Autodesk Inventor part; units mm, degrees
(part 4 of 4)
  line L1587 (9.162058, 31.05913) -> (9.162058, 29.329968)
  line L1588 (9.162058, 29.329968) -> (12.322051, 29.331634)
  line L1589 (12.322051, 29.331634) -> (15.482864, 29.334134)
  line L1590 (15.482864, 29.334134) -> (15.485364, 31.06163)
  line L1591 (15.485364, 31.06163) -> (15.48703, 32.788291)
  line L1592 (15.48703, 32.788291) -> (15.003699, 32.788291)
  line L1593 (15.003699, 32.788291) -> (14.520368, 32.788291)
  line L1594 (14.520368, 32.788291) -> (14.520368, 31.559128)
  line L1595 (14.520368, 31.559128) -> (14.520368, 30.329965)
  line L1596 (14.520368, 30.329965) -> (13.674536, 30.329965)
  line L1597 (13.674536, 30.329965) -> (12.828705, 30.329965)
  line L1598 (12.828705, 30.329965) -> (12.827038, 31.386628)
  line L1599 (12.827038, 31.386628) -> (12.824538, 32.442459)
  line L1600 (12.824538, 32.442459) -> (12.345374, 32.442459)
  line L1601 (12.345374, 32.442459) -> (11.86621, 32.442459)
  line L1602 (11.86621, 32.442459) -> (11.86371, 31.386628)
  line L1603 (11.86371, 31.386628) -> (11.862043, 30.329965)
  line L1604 (11.862043, 30.329965) -> (10.99538, 30.329965)
  line L1605 (10.99538, 30.329965) -> (10.128717, 30.329965)
  line L1606 (10.128717, 30.329965) -> (10.128717, 31.559128)
  line L1607 (10.128717, 31.559128) -> (10.128717, 32.788291)
  line L1608 (10.128717, 32.788291) -> (9.645386, 32.788291)
  line L1609 (9.645386, 32.788291) -> (9.162055, 32.788291)
  line L1610 (9.162055, 32.788291) -> (9.162055, 31.059129)
  line L1611 (9.162055, 31.059129) -> (9.162058, 31.05913)
  line L1612 (9.163727, 35.106681) -> (9.16206, 33.188354)
  line L1613 (9.16206, 33.188354) -> (9.641225, 33.188354)
  line L1614 (9.641225, 33.188354) -> (10.120389, 33.188354)
  line L1615 (10.120389, 33.188354) -> (10.120389, 33.90085)
  line L1616 (10.120389, 33.90085) -> (10.120389, 34.613346)
  line L1617 (10.120389, 34.613346) -> (12.803713, 34.613346)
  line L1618 (12.803713, 34.613346) -> (15.487036, 34.613346)
  line L1619 (15.487036, 34.613346) -> (15.48537, 35.111679)
  line L1620 (15.48537, 35.111679) -> (15.48287, 35.609177)
  line L1621 (15.48287, 35.609177) -> (12.802044, 35.611677)
  line L1622 (12.802044, 35.611677) -> (10.120386, 35.613344)
  line L1623 (10.120386, 35.613344) -> (10.120386, 36.321676)
  line L1624 (10.120386, 36.321676) -> (10.120386, 37.030009)
  line L1625 (10.120386, 37.030009) -> (9.643722, 37.028342)
  line L1626 (9.643722, 37.028342) -> (9.166224, 37.025842)
  line L1627 (9.166224, 37.025842) -> (9.163724, 35.106681)
  line L1628 (9.163724, 35.106681) -> (9.163727, 35.106681)
  line L1629 (5.977339, 133.568916) -> (5.975994, 133.167035)
  line L1630 (5.975994, 133.167035) -> (5.984059, 133.164347)
  line L1631 (5.984059, 133.164347) -> (5.992795, 133.160986)
  line L1632 (5.992795, 133.160986) -> (8.5331, 133.16233)
  line L1633 (8.5331, 133.16233) -> (11.073405, 133.164347)
  line L1634 (11.073405, 133.164347) -> (11.075421, 134.540013)
  line L1635 (11.075421, 134.540013) -> (11.076765, 135.916353)
  line L1636 (11.076765, 135.916353) -> (10.686982, 135.916353)
  line L1637 (10.686982, 135.916353) -> (10.297199, 135.916353)
  line L1638 (10.297199, 135.916353) -> (10.297199, 134.945255)
  line L1639 (10.297199, 134.945255) -> (10.297199, 133.974157)
  line L1640 (10.297199, 133.974157) -> (8.138603, 133.972813)
  line L1641 (8.138603, 133.972813) -> (5.979336, 133.970797)
  line L1642 (5.979336, 133.970797) -> (5.97732, 133.568915)
  line L1643 (5.97732, 133.568915) -> (5.977339, 133.568916)
  line L1644 (5.977339, 136.912318) -> (5.975994, 136.507076)
  line L1645 (5.975994, 136.507076) -> (5.984059, 136.504388)
  line L1646 (5.984059, 136.504388) -> (5.992795, 136.501028)
  line L1647 (5.992795, 136.501028) -> (8.5331, 136.502372)
  line L1648 (8.5331, 136.502372) -> (11.073405, 136.504388)
  line L1649 (11.073405, 136.504388) -> (11.073405, 136.910974)
  line L1650 (11.073405, 136.910974) -> (11.073405, 137.317559)
  line L1651 (11.073405, 137.317559) -> (8.526369, 137.317559)
  line L1652 (8.526369, 137.317559) -> (5.979333, 137.317559)
  line L1653 (5.979333, 137.317559) -> (5.977317, 136.912317)
  line L1654 (5.977317, 136.912317) -> (5.977339, 136.912318)
  line L1655 (5.975992, 138.590496) -> (5.975992, 138.201383)
  line L1656 (5.975992, 138.201383) -> (8.523028, 138.201383)
  line L1657 (8.523028, 138.201383) -> (11.070064, 138.201383)
  line L1658 (11.070064, 138.201383) -> (11.070064, 138.584446)
  line L1659 (11.070064, 138.584446) -> (11.070064, 138.967508)
  line L1660 (11.070064, 138.967508) -> (9.334855, 138.968852)
  line L1661 (9.334855, 138.968852) -> (7.598974, 138.970868)
  line L1662 (7.598974, 138.970868) -> (9.334855, 139.790758)
  line L1663 (9.334855, 139.790758) -> (11.070064, 140.609976)
  line L1664 (11.070064, 140.609976) -> (11.070064, 141.001776)
  line L1665 (11.070064, 141.001776) -> (11.070064, 141.393576)
  line L1666 (11.070064, 141.393576) -> (8.523028, 141.393576)
  line L1667 (8.523028, 141.393576) -> (5.975992, 141.393576)
  line L1668 (5.975992, 141.393576) -> (5.977336, 141.00917)
  line L1669 (5.977336, 141.00917) -> (5.979353, 140.624091)
  line L1670 (5.979353, 140.624091) -> (7.755557, 140.620731)
  line L1671 (7.755557, 140.620731) -> (9.531088, 140.617371)
  line L1672 (9.531088, 140.617371) -> (7.75354, 139.798152)
  line L1673 (7.75354, 139.798152) -> (5.975992, 138.978933)
  line L1674 (5.975992, 138.978933) -> (5.975992, 138.590494)
  line L1675 (5.975992, 138.590494) -> (5.975992, 138.590496)
  line L1676 (5.975992, 143.705294) -> (5.975992, 142.313499)
  line L1677 (5.975992, 142.313499) -> (5.984057, 142.31081)
  line L1678 (5.984057, 142.31081) -> (5.992793, 142.30745)
  line L1679 (5.992793, 142.30745) -> (8.533098, 142.308794)
  line L1680 (8.533098, 142.308794) -> (11.073403, 142.31081)
  line L1681 (11.073403, 142.31081) -> (11.075419, 143.703952)
  line L1682 (11.075419, 143.703952) -> (11.076763, 145.096421)
  line L1683 (11.076763, 145.096421) -> (10.68698, 145.096421)
  line L1684 (10.68698, 145.096421) -> (10.297197, 145.096421)
  line L1685 (10.297197, 145.096421) -> (10.297197, 144.108521)
  line L1686 (10.297197, 144.108521) -> (10.297197, 143.120621)
  line L1687 (10.297197, 143.120621) -> (9.615074, 143.120621)
  line L1688 (9.615074, 143.120621) -> (8.932952, 143.120621)
  line L1689 (8.932952, 143.120621) -> (8.932952, 143.970751)
  line L1690 (8.932952, 143.970751) -> (8.932952, 144.820882)
  line L1691 (8.932952, 144.820882) -> (8.543169, 144.820882)
  line L1692 (8.543169, 144.820882) -> (8.153386, 144.820882)
  line L1693 (8.153386, 144.820882) -> (8.153386, 143.970751)
  line L1694 (8.153386, 143.970751) -> (8.153386, 143.120621)
  line L1695 (8.153386, 143.120621) -> (7.454464, 143.120621)
  line L1696 (7.454464, 143.120621) -> (6.755542, 143.120621)
  line L1697 (6.755542, 143.120621) -> (6.755542, 144.108521)
  line L1698 (6.755542, 144.108521) -> (6.755542, 145.096421)
  line L1699 (6.755542, 145.096421) -> (6.365759, 145.096421)
  line L1700 (6.365759, 145.096421) -> (5.975976, 145.096421)
  line L1701 (5.975976, 145.096421) -> (5.975976, 143.705296)
  line L1702 (5.975976, 143.705296) -> (5.975992, 143.705294)
  line L1703 (5.977339, 148.867844) -> (5.975994, 147.488817)
  line L1704 (5.975994, 147.488817) -> (8.524376, 147.490161)
  line L1705 (8.524376, 147.490161) -> (11.073419, 147.492177)
  line L1706 (11.073419, 147.492177) -> (11.075435, 147.893386)
  line L1707 (11.075435, 147.893386) -> (11.076779, 148.295267)
  line L1708 (11.076779, 148.295267) -> (10.025036, 148.295267)
  line L1709 (10.025036, 148.295267) -> (8.973293, 148.295267)
  line L1710 (8.973293, 148.295267) -> (8.973293, 149.131958)
  line L1711 (8.973293, 149.131958) -> (8.973293, 149.968649)
  line L1712 (8.973293, 149.968649) -> (8.58687, 149.968649)
  line L1713 (8.58687, 149.968649) -> (8.200447, 149.968649)
  line L1714 (8.200447, 149.968649) -> (8.200447, 149.131958)
  line L1715 (8.200447, 149.131958) -> (8.200447, 148.295267)
  line L1716 (8.200447, 148.295267) -> (7.474642, 148.295267)
  line L1717 (7.474642, 148.295267) -> (6.748837, 148.295267)
  line L1718 (6.748837, 148.295267) -> (6.748837, 149.273086)
  line L1719 (6.748837, 149.273086) -> (6.748837, 150.250904)
  line L1720 (6.748837, 150.250904) -> (6.364431, 150.24956)
  line L1721 (6.364431, 150.24956) -> (5.979352, 150.247544)
  line L1722 (5.979352, 150.247544) -> (5.977336, 148.867844)
  line L1723 (5.977336, 148.867844) -> (5.977339, 148.867844)
  line L1724 (5.975992, 155.076112) -> (5.975992, 154.672887)
  line L1725 (5.975992, 154.672887) -> (8.526381, 154.672887)
  line L1726 (8.526381, 154.672887) -> (11.07677, 154.672887)
  line L1727 (11.07677, 154.672887) -> (11.075425, 156.049227)
  line L1728 (11.075425, 156.049227) -> (11.073409, 157.424893)
  line L1729 (11.073409, 157.424893) -> (10.686986, 157.424893)
  line L1730 (10.686986, 157.424893) -> (10.300564, 157.424893)
  line L1731 (10.300564, 157.424893) -> (10.298547, 156.452449)
  line L1732 (10.298547, 156.452449) -> (10.297203, 155.479335)
  line L1733 (10.297203, 155.479335) -> (8.136593, 155.479335)
  line L1734 (8.136593, 155.479335) -> (5.975983, 155.479335)
  line L1735 (5.975983, 155.479335) -> (5.975983, 155.07611)
  line L1736 (5.975983, 155.07611) -> (5.975992, 155.076112)
  line L1737 (5.975992, 158.449994) -> (5.975992, 158.046769)
  line L1738 (5.975992, 158.046769) -> (8.526381, 158.046769)
  line L1739 (8.526381, 158.046769) -> (11.07677, 158.046769)
  line L1740 (11.07677, 158.046769) -> (11.075425, 159.423109)
  line L1741 (11.075425, 159.423109) -> (11.073409, 160.798775)
  line L1742 (11.073409, 160.798775) -> (10.686986, 160.798775)
  line L1743 (10.686986, 160.798775) -> (10.300564, 160.798775)
  line L1744 (10.300564, 160.798775) -> (10.298547, 159.826331)
  line L1745 (10.298547, 159.826331) -> (10.297203, 158.853217)
  line L1746 (10.297203, 158.853217) -> (8.136593, 158.853217)
  line L1747 (8.136593, 158.853217) -> (5.975983, 158.853217)
  line L1748 (5.975983, 158.853217) -> (5.975983, 158.449992)
  line L1749 (5.975983, 158.449992) -> (5.975992, 158.449994)
  line L1750 (5.975992, 165.199282) -> (5.975992, 164.785976)
  line L1751 (5.975992, 164.785976) -> (5.990777, 164.789336)
  line L1752 (5.990777, 164.789336) -> (6.006234, 164.793368)
  line L1753 (6.006234, 164.793368) -> (8.524372, 165.260436)
  line L1754 (8.524372, 165.260436) -> (11.043181, 165.728177)
  line L1755 (11.043181, 165.728177) -> (11.059982, 165.732209)
  line L1756 (11.059982, 165.732209) -> (11.076783, 165.736242)
  line L1757 (11.076783, 165.736242) -> (11.076783, 166.134763)
  line L1758 (11.076783, 166.134763) -> (11.076783, 166.533283)
  line L1759 (11.076783, 166.533283) -> (11.064686, 166.535972)
  line L1760 (11.064686, 166.535972) -> (11.053262, 166.53866)
  line L1761 (11.053262, 166.53866) -> (9.337543, 166.917691)
  line L1762 (9.337543, 166.917691) -> (7.621823, 167.297393)
  line L1763 (7.621823, 167.297393) -> (7.677603, 167.308818)
  line L1764 (7.677603, 167.308818) -> (7.733382, 167.320915)
  line L1765 (7.733382, 167.320915) -> (9.402731, 167.670376)
  line L1766 (9.402731, 167.670376) -> (11.07208, 168.019836)
  line L1767 (11.07208, 168.019836) -> (11.074768, 168.021853)
  line L1768 (11.074768, 168.021853) -> (11.076784, 168.024541)
  line L1769 (11.076784, 168.024541) -> (11.07544, 168.423732)
  line L1770 (11.07544, 168.423732) -> (11.073424, 168.822924)
  line L1771 (11.073424, 168.822924) -> (8.529741, 169.294025)
  line L1772 (8.529741, 169.294025) -> (5.986058, 169.765126)
  line L1773 (5.986058, 169.765126) -> (5.981354, 169.762438)
  line L1774 (5.981354, 169.762438) -> (5.975978, 169.75975)
  line L1775 (5.975978, 169.75975) -> (5.975978, 169.350477)
  line L1776 (5.975978, 169.350477) -> (5.975978, 168.941878)
  line L1777 (5.975978, 168.941878) -> (5.994795, 168.937846)
  line L1778 (5.994795, 168.937846) -> (6.01294, 168.933813)
  line L1779 (6.01294, 168.933813) -> (7.829467, 168.658277)
  line L1780 (7.829467, 168.658277) -> (9.64532, 168.38274)
  line L1781 (9.64532, 168.38274) -> (9.660105, 168.381396)
  line L1782 (9.660105, 168.381396) -> (9.675562, 168.37938)
  line L1783 (9.675562, 168.37938) -> (7.825434, 167.979515)
  line L1784 (7.825434, 167.979515) -> (5.975978, 167.579651)
  line L1785 (5.975978, 167.579651) -> (5.975978, 167.27656)
  line L1786 (5.975978, 167.27656) -> (5.975978, 166.972796)
  line L1787 (5.975978, 166.972796) -> (5.994795, 166.969436)
  line L1788 (5.994795, 166.969436) -> (6.012941, 166.965404)
  line L1789 (6.012941, 166.965404) -> (7.82073, 166.574947)
  line L1790 (7.82073, 166.574947) -> (9.628519, 166.184491)
  line L1791 (9.628519, 166.184491) -> (9.650696, 166.179787)
  line L1792 (9.650696, 166.179787) -> (9.672874, 166.175082)
  line L1793 (9.672874, 166.175082) -> (7.863068, 165.900219)
  line L1794 (7.863068, 165.900219) -> (6.053262, 165.625355)
  line L1795 (6.053262, 165.625355) -> (6.014956, 165.619307)
  line L1796 (6.014956, 165.619307) -> (5.975977, 165.612587)
  line L1797 (5.975977, 165.612587) -> (5.975977, 165.19928)
  line L1798 (5.975977, 165.19928) -> (5.975992, 165.199282)
  line L1799 (5.975992, 171.692538) -> (5.975992, 170.298053)
  line L1800 (5.975992, 170.298053) -> (8.526381, 170.298053)
  line L1801 (8.526381, 170.298053) -> (11.07677, 170.298053)
  line L1802 (11.07677, 170.298053) -> (11.07677, 171.692538)
  line L1803 (11.07677, 171.692538) -> (11.07677, 173.087023)
  line L1804 (11.07677, 173.087023) -> (10.686986, 173.087023)
  line L1805 (10.686986, 173.087023) -> (10.297203, 173.087023)
  line L1806 (10.297203, 173.087023) -> (10.297203, 172.095763)
  line L1807 (10.297203, 172.095763) -> (10.297203, 171.104503)
  line L1808 (10.297203, 171.104503) -> (9.615081, 171.104503)
  line L1809 (9.615081, 171.104503) -> (8.932959, 171.104503)
  line L1810 (8.932959, 171.104503) -> (8.932959, 171.954633)
  line L1811 (8.932959, 171.954633) -> (8.932959, 172.804763)
  line L1812 (8.932959, 172.804763) -> (8.543175, 172.804763)
  line L1813 (8.543175, 172.804763) -> (8.153392, 172.804763)
  line L1814 (8.153392, 172.804763) -> (8.153392, 171.954633)
  line L1815 (8.153392, 171.954633) -> (8.153392, 171.104503)
  line L1816 (8.153392, 171.104503) -> (7.45447, 171.104503)
  line L1817 (7.45447, 171.104503) -> (6.755549, 171.104503)
  line L1818 (6.755549, 171.104503) -> (6.755549, 172.095763)
  line L1819 (6.755549, 172.095763) -> (6.755549, 173.087023)
  line L1820 (6.755549, 173.087023) -> (6.365765, 173.087023)
  line L1821 (6.365765, 173.087023) -> (5.975982, 173.087023)
  line L1822 (5.975982, 173.087023) -> (5.975982, 171.692538)
  line L1823 (5.975982, 171.692538) -> (5.975992, 171.692538)
  line L1824 (5.977339, 174.71463) -> (5.975994, 173.79259)
  line L1825 (5.975994, 173.79259) -> (8.52303, 173.79259)
  line L1826 (8.52303, 173.79259) -> (11.070066, 173.79259)
  line L1827 (11.070066, 173.79259) -> (11.070066, 174.195815)
  line L1828 (11.070066, 174.195815) -> (11.070066, 174.59904)
  line L1829 (11.070066, 174.59904) -> (10.008242, 174.59904)
  line L1830 (10.008242, 174.59904) -> (8.946418, 174.59904)
  line L1831 (8.946418, 174.59904) -> (8.947762, 174.909522)
  line L1832 (8.947762, 174.909522) -> (8.949778, 175.220677)
  line L1833 (8.949778, 175.220677) -> (10.009585, 175.660191)
  line L1834 (10.009585, 175.660191) -> (11.070066, 176.100378)
  line L1835 (11.070066, 176.100378) -> (11.070066, 176.562742)
  line L1836 (11.070066, 176.562742) -> (11.070066, 177.025105)
  line L1837 (11.070066, 177.025105) -> (11.03512, 177.009649)
  line L1838 (11.03512, 177.009649) -> (10.999502, 176.99352)
  line L1839 (10.999502, 176.99352) -> (9.924909, 176.521748)
  line L1840 (9.924909, 176.521748) -> (8.850316, 176.049976)
  line L1841 (8.850316, 176.049976) -> (8.846284, 176.057368)
  line L1842 (8.846284, 176.057368) -> (8.842252, 176.064088)
  line L1843 (8.842252, 176.064088) -> (8.82209, 176.113148)
  line L1844 (8.82209, 176.113148) -> (8.801257, 176.161535)
  line L1845 (8.801257, 176.161535) -> (8.777736, 176.207905)
  line L1846 (8.777736, 176.207905) -> (8.754214, 176.254276)
  line L1847 (8.754214, 176.254276) -> (8.710532, 176.318792)
  line L1848 (8.710532, 176.318792) -> (8.667521, 176.382636)
  line L1849 (8.667521, 176.382636) -> (8.617118, 176.43976)
  line L1850 (8.617118, 176.43976) -> (8.566715, 176.496883)
  line L1851 (8.566715, 176.496883) -> (8.502871, 176.549302)
  line L1852 (8.502871, 176.549302) -> (8.439027, 176.601722)
  line L1853 (8.439027, 176.601722) -> (8.394, 176.631963)
  line L1854 (8.394, 176.631963) -> (8.348302, 176.662205)
  line L1855 (8.348302, 176.662205) -> (8.259592, 176.705216)
  line L1856 (8.259592, 176.705216) -> (8.170211, 176.748226)
  line L1857 (8.170211, 176.748226) -> (8.089566, 176.773764)
  line L1858 (8.089566, 176.773764) -> (8.008921, 176.799302)
  line L1859 (8.008921, 176.799302) -> (7.924916, 176.815431)
  line L1860 (7.924916, 176.815431) -> (7.840911, 176.83156)
  line L1861 (7.840911, 176.83156) -> (7.753545, 176.838952)
  line L1862 (7.753545, 176.838952) -> (7.66618, 176.845672)
  line L1863 (7.66618, 176.845672) -> (7.383922, 176.842312)
  line L1864 (7.383922, 176.842312) -> (7.101665, 176.83828)
  line L1865 (7.101665, 176.83828) -> (7.023708, 176.824167)
  line L1866 (7.023708, 176.824167) -> (6.945752, 176.809382)
  line L1867 (6.945752, 176.809382) -> (6.88258, 176.792581)
  line L1868 (6.88258, 176.792581) -> (6.819408, 176.775108)
  line L1869 (6.819408, 176.775108) -> (6.765645, 176.756291)
  line L1870 (6.765645, 176.756291) -> (6.711882, 176.737474)
  line L1871 (6.711882, 176.737474) -> (6.627876, 176.693791)
  line L1872 (6.627876, 176.693791) -> (6.543871, 176.650109)
  line L1873 (6.543871, 176.650109) -> (6.486748, 176.61113)
  line L1874 (6.486748, 176.61113) -> (6.429624, 176.57148)
  line L1875 (6.429624, 176.57148) -> (6.342259, 176.484114)
  line L1876 (6.342259, 176.484114) -> (6.254893, 176.396749)
  line L1877 (6.254893, 176.396749) -> (6.20449, 176.319465)
  line L1878 (6.20449, 176.319465) -> (6.154087, 176.24218)
  line L1879 (6.154087, 176.24218) -> (6.123174, 176.178336)
  line L1880 (6.123174, 176.178336) -> (6.09226, 176.114492)
  line L1881 (6.09226, 176.114492) -> (6.074787, 176.067449)
  line L1882 (6.074787, 176.067449) -> (6.057314, 176.020406)
  line L1883 (6.057314, 176.020406) -> (6.039841, 175.963283)
  line L1884 (6.039841, 175.963283) -> (6.022368, 175.906159)
  line L1885 (6.022368, 175.906159) -> (6.008927, 175.835595)
  line L1886 (6.008927, 175.835595) -> (5.995486, 175.765031)
  line L1887 (5.995486, 175.765031) -> (5.987421, 175.701187)
  line L1888 (5.987421, 175.701187) -> (5.979357, 175.637343)
  line L1889 (5.979357, 175.637343) -> (5.977341, 174.714632)
  line L1890 (5.977341, 174.714632) -> (5.977339, 174.71463)
  line L1891 (6.750184, 175.097693) -> (6.752872, 175.597018)
  line L1892 (6.752872, 175.597018) -> (6.764297, 175.637341)
  line L1893 (6.764297, 175.637341) -> (6.775722, 175.677663)
  line L1894 (6.775722, 175.677663) -> (6.802603, 175.731427)
  line L1895 (6.802603, 175.731427) -> (6.828813, 175.78519)
  line L1896 (6.828813, 175.78519) -> (6.863759, 175.825512)
  line L1897 (6.863759, 175.825512) -> (6.899377, 175.865835)
  line L1898 (6.899377, 175.865835) -> (6.929619, 175.890028)
  line L1899 (6.929619, 175.890028) -> (6.960533, 175.91355)
  line L1900 (6.960533, 175.91355) -> (6.997495, 175.935055)
  line L1901 (6.997495, 175.935055) -> (7.034457, 175.955888)
  line L1902 (7.034457, 175.955888) -> (7.096957, 175.976049)
  line L1903 (7.096957, 175.976049) -> (7.158785, 175.996883)
  line L1904 (7.158785, 175.996883) -> (7.211204, 176.004275)
  line L1905 (7.211204, 176.004275) -> (7.262951, 176.011668)
  line L1906 (7.262951, 176.011668) -> (7.498166, 176.008307)
  line L1907 (7.498166, 176.008307) -> (7.73338, 176.005619)
  line L1908 (7.73338, 176.005619) -> (7.790503, 175.991506)
  line L1909 (7.790503, 175.991506) -> (7.847627, 175.976721)
  line L1910 (7.847627, 175.976721) -> (7.910127, 175.945136)
  line L1911 (7.910127, 175.945136) -> (7.973299, 175.91355)
  line L1912 (7.973299, 175.91355) -> (8.025046, 175.863147)
  line L1913 (8.025046, 175.863147) -> (8.076121, 175.812072)
  line L1914 (8.076121, 175.812072) -> (8.101659, 175.768389)
  line L1915 (8.101659, 175.768389) -> (8.127196, 175.724706)
  line L1916 (8.127196, 175.724706) -> (8.142653, 175.674303)
  line L1917 (8.142653, 175.674303) -> (8.158782, 175.6239)
  line L1918 (8.158782, 175.6239) -> (8.166175, 175.565433)
  line L1919 (8.166175, 175.565433) -> (8.173567, 175.506293)
  line L1920 (8.173567, 175.506293) -> (8.173567, 175.052664)
  line L1921 (8.173567, 175.052664) -> (8.173567, 174.599036)
  line L1922 (8.173567, 174.599036) -> (7.461204, 174.599036)
  line L1923 (7.461204, 174.599036) -> (6.748167, 174.599036)
  line L1924 (6.748167, 174.599036) -> (6.750183, 175.097691)
  line L1925 (6.750183, 175.097691) -> (6.750184, 175.097693)
  line L1926 (5.977339, 179.835524) -> (5.975994, 179.430955)
  line L1927 (5.975994, 179.430955) -> (8.524376, 179.432299)
  line L1928 (8.524376, 179.432299) -> (11.073419, 179.434316)
  line L1929 (11.073419, 179.434316) -> (11.075435, 180.809982)
  line L1930 (11.075435, 180.809982) -> (11.076779, 182.186322)
  line L1931 (11.076779, 182.186322) -> (10.686996, 182.186322)
  line L1932 (10.686996, 182.186322) -> (10.297212, 182.186322)
  line L1933 (10.297212, 182.186322) -> (10.297212, 181.215224)
  line L1934 (10.297212, 181.215224) -> (10.297212, 180.244126)
  line L1935 (10.297212, 180.244126) -> (8.138616, 180.242782)
  line L1936 (8.138616, 180.242782) -> (5.97935, 180.240766)
  line L1937 (5.97935, 180.240766) -> (5.977333, 179.835524)
  line L1938 (5.977333, 179.835524) -> (5.977339, 179.835524)
  line L1939 (5.975992, 184.371202) -> (5.975992, 184.064751)
  line L1940 (5.975992, 184.064751) -> (8.518329, 183.289215)
  line L1941 (8.518329, 183.289215) -> (11.05998, 182.51368)
  line L1942 (11.05998, 182.51368) -> (11.066701, 182.513008)
  line L1943 (11.066701, 182.513008) -> (11.073421, 182.512336)
  line L1944 (11.073421, 182.512336) -> (11.075437, 182.937064)
  line L1945 (11.075437, 182.937064) -> (11.076781, 183.361793)
  line L1946 (11.076781, 183.361793) -> (11.051916, 183.368513)
  line L1947 (11.051916, 183.368513) -> (11.026378, 183.375234)
  line L1948 (11.026378, 183.375234) -> (10.571406, 183.498217)
  line L1949 (10.571406, 183.498217) -> (10.115763, 183.621201)
  line L1950 (10.115763, 183.621201) -> (10.117779, 184.373213)
  line L1951 (10.117779, 184.373213) -> (10.119123, 185.125226)
  line L1952 (10.119123, 185.125226) -> (10.596272, 185.254258)
  line L1953 (10.596272, 185.254258) -> (11.073421, 185.383962)
  line L1954 (11.073421, 185.383962) -> (11.075437, 185.80869)
  line L1955 (11.075437, 185.80869) -> (11.076781, 186.233419)
  line L1956 (11.076781, 186.233419) -> (11.058636, 186.228715)
  line L1957 (11.058636, 186.228715) -> (11.040491, 186.224682)
  line L1958 (11.040491, 186.224682) -> (8.565365, 185.468636)
  line L1959 (8.565365, 185.468636) -> (6.090239, 184.713263)
  line L1960 (6.090239, 184.713263) -> (6.033116, 184.69579)
  line L1961 (6.033116, 184.69579) -> (5.975992, 184.678317)
  line L1962 (5.975992, 184.678317) -> (5.975992, 184.371195)
  line L1963 (5.975992, 184.371195) -> (5.975992, 184.371202)
  line L1964 (8.328807, 184.639347) -> (9.312676, 184.906819)
  line L1965 (9.312676, 184.906819) -> (9.330821, 184.911524)
  line L1966 (9.330821, 184.911524) -> (9.349638, 184.916228)
  line L1967 (9.349638, 184.916228) -> (9.349638, 184.374563)
  line L1968 (9.349638, 184.374563) -> (9.349638, 183.832898)
  line L1969 (9.349638, 183.832898) -> (9.342246, 183.832898)
  line L1970 (9.342246, 183.832898) -> (9.334853, 183.832898)
  line L1971 (9.334853, 183.832898) -> (8.362409, 184.094993)
  line L1972 (8.362409, 184.094993) -> (7.390638, 184.357761)
  line L1973 (7.390638, 184.357761) -> (7.367789, 184.365153)
  line L1974 (7.367789, 184.365153) -> (7.344268, 184.372546)
  line L1975 (7.344268, 184.372546) -> (8.328807, 184.639345)
  line L1976 (8.328807, 184.639345) -> (8.328807, 184.639347)
  line L1977 (5.977339, 187.671678) -> (5.975994, 186.783239)
  line L1978 (5.975994, 186.783239) -> (8.526383, 186.783239)
  line L1979 (8.526383, 186.783239) -> (11.076772, 186.783239)
  line L1980 (11.076772, 186.783239) -> (11.076772, 187.186464)
  line L1981 (11.076772, 187.186464) -> (11.076772, 187.589689)
  line L1982 (11.076772, 187.589689) -> (10.089545, 187.589689)
  line L1983 (10.089545, 187.589689) -> (9.102318, 187.589689)
  line L1984 (9.102318, 187.589689) -> (9.098958, 188.105817)
  line L1985 (9.098958, 188.105817) -> (9.095597, 188.621272)
  line L1986 (9.095597, 188.621272) -> (9.084845, 188.695869)
  line L1987 (9.084845, 188.695869) -> (9.07342, 188.769793)
  line L1988 (9.07342, 188.769793) -> (9.057291, 188.845062)
  line L1989 (9.057291, 188.845062) -> (9.04049, 188.92033)
  line L1990 (9.04049, 188.92033) -> (9.014952, 188.992911)
  line L1991 (9.014952, 188.992911) -> (8.989415, 189.064819)
  line L1992 (8.989415, 189.064819) -> (8.962533, 189.122615)
  line L1993 (8.962533, 189.122615) -> (8.936324, 189.18041)
  line L1994 (8.936324, 189.18041) -> (8.896001, 189.245598)
  line L1995 (8.896001, 189.245598) -> (8.855679, 189.310786)
  line L1996 (8.855679, 189.310786) -> (8.811996, 189.365894)
  line L1997 (8.811996, 189.365894) -> (8.768313, 189.420329)
  line L1998 (8.768313, 189.420329) -> (8.715894, 189.471404)
  line L1999 (8.715894, 189.471404) -> (8.663475, 189.521807)
  line L2000 (8.663475, 189.521807) -> (8.632561, 189.546)
  line L2001 (8.632561, 189.546) -> (8.602319, 189.570866)
  line L2002 (8.602319, 189.570866) -> (8.543852, 189.609172)
  line L2003 (8.543852, 189.609172) -> (8.486056, 189.646806)
  line L2004 (8.486056, 189.646806) -> (8.417508, 189.680408)
  line L2005 (8.417508, 189.680408) -> (8.34896, 189.71401)
  line L2006 (8.34896, 189.71401) -> (8.256218, 189.744252)
  line L2007 (8.256218, 189.744252) -> (8.163476, 189.774494)
  line L2008 (8.163476, 189.774494) -> (8.092912, 189.788607)
  line L2009 (8.092912, 189.788607) -> (8.022348, 189.802047)
  line L2010 (8.022348, 189.802047) -> (7.961864, 189.810112)
  line L2011 (7.961864, 189.810112) -> (7.90138, 189.817504)
  line L2012 (7.90138, 189.817504) -> (7.525039, 189.816832)
  line L2013 (7.525039, 189.816832) -> (7.148697, 189.815488)
  line L2014 (7.148697, 189.815488) -> (7.078133, 189.804063)
  line L2015 (7.078133, 189.804063) -> (7.007569, 189.791967)
  line L2016 (7.007569, 189.791967) -> (6.96523, 189.78323)
  line L2017 (6.96523, 189.78323) -> (6.923564, 189.773822)
  line L2018 (6.923564, 189.773822) -> (6.864424, 189.756349)
  line L2019 (6.864424, 189.756349) -> (6.805957, 189.739548)
  line L2020 (6.805957, 189.739548) -> (6.751521, 189.71737)
  line L2021 (6.751521, 189.71737) -> (6.697086, 189.695193)
  line L2022 (6.697086, 189.695193) -> (6.638619, 189.665623)
  line L2023 (6.638619, 189.665623) -> (6.579479, 189.636053)
  line L2024 (6.579479, 189.636053) -> (6.514963, 189.59237)
  line L2025 (6.514963, 189.59237) -> (6.449775, 189.548688)
  line L2026 (6.449775, 189.548688) -> (6.399372, 189.504333)
  line L2027 (6.399372, 189.504333) -> (6.348969, 189.459978)
  line L2028 (6.348969, 189.459978) -> (6.308646, 189.414951)
  line L2029 (6.308646, 189.414951) -> (6.268324, 189.370597)
  line L2030 (6.268324, 189.370597) -> (6.23069, 189.319522)
  line L2031 (6.23069, 189.319522) -> (6.193727, 189.268446)
  line L2032 (6.193727, 189.268446) -> (6.158781, 189.207291)
  line L2033 (6.158781, 189.207291) -> (6.123835, 189.145463)
  line L2034 (6.123835, 189.145463) -> (6.094265, 189.074899)
  line L2035 (6.094265, 189.074899) -> (6.064695, 189.004334)
  line L2036 (6.064695, 189.004334) -> (6.04655, 188.945867)
  line L2037 (6.04655, 188.945867) -> (6.028405, 188.887399)
  line L2038 (6.028405, 188.887399) -> (6.011604, 188.801378)
  line L2039 (6.011604, 188.801378) -> (5.994803, 188.715357)
  line L2040 (5.994803, 188.715357) -> (5.986739, 188.638073)
  line L2041 (5.986739, 188.638073) -> (5.979346, 188.560788)
  line L2042 (5.979346, 188.560788) -> (5.97733, 187.671679)
  line L2043 (5.97733, 187.671679) -> (5.977339, 187.671678)
  line L2044 (6.750184, 188.072213) -> (6.752872, 188.554066)
  line L2045 (6.752872, 188.554066) -> (6.767657, 188.606486)
  line L2046 (6.767657, 188.606486) -> (6.78177, 188.658905)
  line L2047 (6.78177, 188.658905) -> (6.809324, 188.711324)
  line L2048 (6.809324, 188.711324) -> (6.836205, 188.763071)
  line L2049 (6.836205, 188.763071) -> (6.871152, 188.80205)
  line L2050 (6.871152, 188.80205) -> (6.905426, 188.841028)
  line L2051 (6.905426, 188.841028) -> (6.940372, 188.866566)
  line L2052 (6.940372, 188.866566) -> (6.975318, 188.892775)
  line L2053 (6.975318, 188.892775) -> (7.021688, 188.916297)
  line L2054 (7.021688, 188.916297) -> (7.068059, 188.939146)
  line L2055 (7.068059, 188.939146) -> (7.109726, 188.953259)
  line L2056 (7.109726, 188.953259) -> (7.151392, 188.967372)
  line L2057 (7.151392, 188.967372) -> (7.213892, 188.978796)
  line L2058 (7.213892, 188.978796) -> (7.276392, 188.990221)
  line L2059 (7.276392, 188.990221) -> (7.541847, 188.990893)
  line L2060 (7.541847, 188.990893) -> (7.807302, 188.990893)
  line L2061 (7.807302, 188.990893) -> (7.869802, 188.978796)
  line L2062 (7.869802, 188.978796) -> (7.932974, 188.967372)
  line L2063 (7.932974, 188.967372) -> (7.992114, 188.944522)
  line L2064 (7.992114, 188.944522) -> (8.051925, 188.922345)
  line L2065 (8.051925, 188.922345) -> (8.090904, 188.899496)
  line L2066 (8.090904, 188.899496) -> (8.129882, 188.876646)
  line L2067 (8.129882, 188.876646) -> (8.183645, 188.822883)
  line L2068 (8.183645, 188.822883) -> (8.23808, 188.76912)
  line L2069 (8.23808, 188.76912) -> (8.266306, 188.714013)
  line L2070 (8.266306, 188.714013) -> (8.295204, 188.658905)
  line L2071 (8.295204, 188.658905) -> (8.309317, 188.606486)
  line L2072 (8.309317, 188.606486) -> (8.324102, 188.554067)
  line L2073 (8.324102, 188.554067) -> (8.32679, 188.072213)
  line L2074 (8.32679, 188.072213) -> (8.328806, 187.589687)
  line L2075 (8.328806, 187.589687) -> (7.538485, 187.589687)
  line L2076 (7.538485, 187.589687) -> (6.748164, 187.589687)
  line L2077 (6.748164, 187.589687) -> (6.75018, 188.072213)
  line L2078 (6.75018, 188.072213) -> (6.750184, 188.072213)
  line L2079 (5.975992, 193.28838) -> (5.975992, 191.742686)
  line L2080 (5.975992, 191.742686) -> (6.362415, 191.742686)
  line L2081 (6.362415, 191.742686) -> (6.748838, 191.742686)
  line L2082 (6.748838, 191.742686) -> (6.748838, 192.313922)
  line L2083 (6.748838, 192.313922) -> (6.748838, 192.885158)
  line L2084 (6.748838, 192.885158) -> (8.912809, 192.885158)
  line L2085 (8.912809, 192.885158) -> (11.07678, 192.885158)
  line L2086 (11.07678, 192.885158) -> (11.07678, 193.288383)
  line L2087 (11.07678, 193.288383) -> (11.07678, 193.691608)
  line L2088 (11.07678, 193.691608) -> (8.912809, 193.691608)
  line L2089 (8.912809, 193.691608) -> (6.748838, 193.691608)
  line L2090 (6.748838, 193.691608) -> (6.748838, 194.262843)
  line L2091 (6.748838, 194.262843) -> (6.748838, 194.834079)
  line L2092 (6.748838, 194.834079) -> (6.362415, 194.834079)
  line L2093 (6.362415, 194.834079) -> (5.975992, 194.834079)
  line L2094 (5.975992, 194.834079) -> (5.975992, 193.288385)
  line L2095 (5.975992, 193.288385) -> (5.975992, 193.28838)
  line L2096 (5.975992, 195.737956) -> (5.975992, 195.331371)
  line L2097 (5.975992, 195.331371) -> (8.526381, 195.331371)
  line L2098 (8.526381, 195.331371) -> (11.07677, 195.331371)
  line L2099 (11.07677, 195.331371) -> (11.07677, 195.737956)
  line L2100 (11.07677, 195.737956) -> (11.07677, 196.144541)
  line L2101 (11.07677, 196.144541) -> (8.526381, 196.144541)
  line L2102 (8.526381, 196.144541) -> (5.975992, 196.144541)
  line L2103 (5.975992, 196.144541) -> (5.975992, 195.737956)
  line L2104 (5.975992, 197.453726) -> (5.975992, 197.031012)
  line L2105 (5.975992, 197.031012) -> (5.984057, 197.028323)
  line L2106 (5.984057, 197.028323) -> (5.992793, 197.024963)
  line L2107 (5.992793, 197.024963) -> (8.533098, 197.026307)
  line L2108 (8.533098, 197.026307) -> (11.073403, 197.028323)
  line L2109 (11.073403, 197.028323) -> (11.073403, 197.404665)
  line L2110 (11.073403, 197.404665) -> (11.073403, 197.781007)
  line L2111 (11.073403, 197.781007) -> (9.416823, 197.784367)
  line L2112 (9.416823, 197.784367) -> (7.760913, 197.787727)
  line L2113 (7.760913, 197.787727) -> (9.040478, 198.234635)
  line L2114 (9.040478, 198.234635) -> (10.320717, 198.681543)
  line L2115 (10.320717, 198.681543) -> (10.320717, 198.96044)
  line L2116 (10.320717, 198.96044) -> (10.320717, 199.239337)
  line L2117 (10.320717, 199.239337) -> (8.98806, 199.692966)
  line L2118 (8.98806, 199.692966) -> (7.655404, 200.146595)
  line L2119 (7.655404, 200.146595) -> (9.366419, 200.148611)
  line L2120 (9.366419, 200.148611) -> (11.076763, 200.149955)
  line L2121 (11.076763, 200.149955) -> (11.076763, 200.519578)
  line L2122 (11.076763, 200.519578) -> (11.076763, 200.889202)
  line L2123 (11.076763, 200.889202) -> (8.526375, 200.889202)
  line L2124 (8.526375, 200.889202) -> (5.975986, 200.889202)
  line L2125 (5.975986, 200.889202) -> (5.97733, 200.471191)
  line L2126 (5.97733, 200.471191) -> (5.979346, 200.05251)
  line L2127 (5.979346, 200.05251) -> (7.563346, 199.508158)
  line L2128 (7.563346, 199.508158) -> (9.148019, 198.963805)
  line L2129 (9.148019, 198.963805) -> (9.148019, 198.960445)
  line L2130 (9.148019, 198.960445) -> (9.148019, 198.956413)
  line L2131 (9.148019, 198.956413) -> (7.670875, 198.454397)
  line L2132 (7.670875, 198.454397) -> (6.194401, 197.951711)
  line L2133 (6.194401, 197.951711) -> (6.084858, 197.914077)
  line L2134 (6.084858, 197.914077) -> (5.975987, 197.876443)
  line L2135 (5.975987, 197.876443) -> (5.975987, 197.453728)
  line L2136 (5.975987, 197.453728) -> (5.975992, 197.453726)
  line L2137 (5.975992, 203.20454) -> (5.975992, 201.810055)
  line L2138 (5.975992, 201.810055) -> (8.526381, 201.810055)
  line L2139 (8.526381, 201.810055) -> (11.07677, 201.810055)
  line L2140 (11.07677, 201.810055) -> (11.07677, 203.20454)
  line L2141 (11.07677, 203.20454) -> (11.07677, 204.599025)
  line L2142 (11.07677, 204.599025) -> (10.686986, 204.599025)
  line L2143 (10.686986, 204.599025) -> (10.297203, 204.599025)
  line L2144 (10.297203, 204.599025) -> (10.297203, 203.607765)
  line L2145 (10.297203, 203.607765) -> (10.297203, 202.616505)
  line L2146 (10.297203, 202.616505) -> (9.615081, 202.616505)
  line L2147 (9.615081, 202.616505) -> (8.932959, 202.616505)
  line L2148 (8.932959, 202.616505) -> (8.932959, 203.466635)
  line L2149 (8.932959, 203.466635) -> (8.932959, 204.316765)
  line L2150 (8.932959, 204.316765) -> (8.543175, 204.316765)
  line L2151 (8.543175, 204.316765) -> (8.153392, 204.316765)
  line L2152 (8.153392, 204.316765) -> (8.153392, 203.466635)
  line L2153 (8.153392, 203.466635) -> (8.153392, 202.616505)
  line L2154 (8.153392, 202.616505) -> (7.45447, 202.616505)
  line L2155 (7.45447, 202.616505) -> (6.755549, 202.616505)
  line L2156 (6.755549, 202.616505) -> (6.755549, 203.607765)
  line L2157 (6.755549, 203.607765) -> (6.755549, 204.599025)
  line L2158 (6.755549, 204.599025) -> (6.365765, 204.599025)
  line L2159 (6.365765, 204.599025) -> (5.975982, 204.599025)
  line L2160 (5.975982, 204.599025) -> (5.975982, 203.20454)
  line L2161 (5.975982, 203.20454) -> (5.975992, 203.20454)
  line L2162 (5.975332, 206.172784) -> (5.976004, 205.304508)
  line L2163 (5.976004, 205.304508) -> (8.52304, 205.304508)
  line L2164 (8.52304, 205.304508) -> (11.070076, 205.304508)
  line L2165 (11.070076, 205.304508) -> (11.070076, 205.707733)
  line L2166 (11.070076, 205.707733) -> (11.070076, 206.110958)
  line L2167 (11.070076, 206.110958) -> (10.008251, 206.110958)
  line L2168 (10.008251, 206.110958) -> (8.946427, 206.110958)
  line L2169 (8.946427, 206.110958) -> (8.947771, 206.42144)
  line L2170 (8.947771, 206.42144) -> (8.949787, 206.732595)
  line L2171 (8.949787, 206.732595) -> (10.009595, 207.172782)
  line L2172 (10.009595, 207.172782) -> (11.070075, 207.612969)
  line L2173 (11.070075, 207.612969) -> (11.070075, 208.074662)
  line L2174 (11.070075, 208.074662) -> (11.070075, 208.537026)
  line L2175 (11.070075, 208.537026) -> (11.031097, 208.519553)
  line L2176 (11.031097, 208.519553) -> (10.992791, 208.502752)
  line L2177 (10.992791, 208.502752) -> (9.921558, 208.032324)
  line L2178 (9.921558, 208.032324) -> (8.850326, 207.561895)
  line L2179 (8.850326, 207.561895) -> (8.849654, 207.563912)
  line L2180 (8.849654, 207.563912) -> (8.84831, 207.565928)
  line L2181 (8.84831, 207.565928) -> (8.826805, 207.614987)
  line L2182 (8.826805, 207.614987) -> (8.805299, 207.663374)
  line L2183 (8.805299, 207.663374) -> (8.779762, 207.713777)
  line L2184 (8.779762, 207.713777) -> (8.754896, 207.764852)
  line L2185 (8.754896, 207.764852) -> (8.711214, 207.829368)
  line L2186 (8.711214, 207.829368) -> (8.667531, 207.894556)
  line L2187 (8.667531, 207.894556) -> (8.617128, 207.95168)
  line L2188 (8.617128, 207.95168) -> (8.566053, 208.008803)
  line L2189 (8.566053, 208.008803) -> (8.514306, 208.053158)
  line L2190 (8.514306, 208.053158) -> (8.462558, 208.096841)
  line L2191 (8.462558, 208.096841) -> (8.39401, 208.141867)
  line L2192 (8.39401, 208.141867) -> (8.32479, 208.187566)
  line L2193 (8.32479, 208.187566) -> (8.246161, 208.224528)
  line L2194 (8.246161, 208.224528) -> (8.166861, 208.261491)
  line L2195 (8.166861, 208.261491) -> (8.105033, 208.281652)
  line L2196 (8.105033, 208.281652) -> (8.042533, 208.302485)
  line L2197 (8.042533, 208.302485) -> (7.965249, 208.319286)
  line L2198 (7.965249, 208.319286) -> (7.887964, 208.336087)
  line L2199 (7.887964, 208.336087) -> (7.82748, 208.344152)
  line L2200 (7.82748, 208.344152) -> (7.766997, 208.352216)
  line L2201 (7.766997, 208.352216) -> (7.434335, 208.351544)
  line L2202 (7.434335, 208.351544) -> (7.101674, 208.3502)
  line L2203 (7.101674, 208.3502) -> (7.039174, 208.339447)
  line L2204 (7.039174, 208.339447) -> (6.977347, 208.328695)
  line L2205 (6.977347, 208.328695) -> (6.902078, 208.309206)
  line L2206 (6.902078, 208.309206) -> (6.826137, 208.289716)
  line L2207 (6.826137, 208.289716) -> (6.769014, 208.269555)
  line L2208 (6.769014, 208.269555) -> (6.71189, 208.249394)
  line L2209 (6.71189, 208.249394) -> (6.627885, 208.205711)
  line L2210 (6.627885, 208.205711) -> (6.54388, 208.162701)
  line L2211 (6.54388, 208.162701) -> (6.500197, 208.132459)
  line L2212 (6.500197, 208.132459) -> (6.456515, 208.102217)
  line L2213 (6.456515, 208.102217) -> (6.406784, 208.059207)
  line L2214 (6.406784, 208.059207) -> (6.357053, 208.016196)
  line L2215 (6.357053, 208.016196) -> (6.305978, 207.961761)
  line L2216 (6.305978, 207.961761) -> (6.254903, 207.906653)
  line L2217 (6.254903, 207.906653) -> (6.2045, 207.830713)
  line L2218 (6.2045, 207.830713) -> (6.154097, 207.7541)
  line L2219 (6.154097, 207.7541) -> (6.123183, 207.690256)
  line L2220 (6.123183, 207.690256) -> (6.092269, 207.626412)
  line L2221 (6.092269, 207.626412) -> (6.070764, 207.569289)
  line L2222 (6.070764, 207.569289) -> (6.04993, 207.512165)
  line L2223 (6.04993, 207.512165) -> (6.032457, 207.450337)
  line L2224 (6.032457, 207.450337) -> (6.014984, 207.38851)
  line L2225 (6.014984, 207.38851) -> (6.000871, 207.302489)
  line L2226 (6.000871, 207.302489) -> (5.986086, 207.216467)
  line L2227 (5.986086, 207.216467) -> (5.98071, 207.129102)
  line L2228 (5.98071, 207.129102) -> (5.974662, 207.041737)
  line L2229 (5.974662, 207.041737) -> (5.975334, 206.172788)
  line L2230 (5.975334, 206.172788) -> (5.975332, 206.172784)
  line L2231 (6.750194, 206.609611) -> (6.752883, 207.108937)
  line L2232 (6.752883, 207.108937) -> (6.764307, 207.149259)
  line L2233 (6.764307, 207.149259) -> (6.775732, 207.189582)
  line L2234 (6.775732, 207.189582) -> (6.802614, 207.244017)
  line L2235 (6.802614, 207.244017) -> (6.828823, 207.298452)
  line L2236 (6.828823, 207.298452) -> (6.867801, 207.341463)
  line L2237 (6.867801, 207.341463) -> (6.906108, 207.384473)
  line L2238 (6.906108, 207.384473) -> (6.932989, 207.405307)
  line L2239 (6.932989, 207.405307) -> (6.960543, 207.425468)
  line L2240 (6.960543, 207.425468) -> (6.997505, 207.446973)
  line L2241 (6.997505, 207.446973) -> (7.034468, 207.467806)
  line L2242 (7.034468, 207.467806) -> (7.096967, 207.487968)
  line L2243 (7.096967, 207.487968) -> (7.158795, 207.508801)
  line L2244 (7.158795, 207.508801) -> (7.211214, 207.516193)
  line L2245 (7.211214, 207.516193) -> (7.262961, 207.523586)
  line L2246 (7.262961, 207.523586) -> (7.501536, 207.520898)
  line L2247 (7.501536, 207.520898) -> (7.740111, 207.518209)
  line L2248 (7.740111, 207.518209) -> (7.793874, 207.502752)
  line L2249 (7.793874, 207.502752) -> (7.847637, 207.487968)
  line L2250 (7.847637, 207.487968) -> (7.910809, 207.457054)
  line L2251 (7.910809, 207.457054) -> (7.973308, 207.42614)
  line L2252 (7.973308, 207.42614) -> (8.025056, 207.375065)
  line L2253 (8.025056, 207.375065) -> (8.076131, 207.32399)
  line L2254 (8.076131, 207.32399) -> (8.101668, 207.280307)
  line L2255 (8.101668, 207.280307) -> (8.127206, 207.236624)
  line L2256 (8.127206, 207.236624) -> (8.142663, 207.186221)
  line L2257 (8.142663, 207.186221) -> (8.158792, 207.135818)
  line L2258 (8.158792, 207.135818) -> (8.166184, 207.077351)
  line L2259 (8.166184, 207.077351) -> (8.173577, 207.018211)
  line L2260 (8.173577, 207.018211) -> (8.173577, 206.564583)
  line L2261 (8.173577, 206.564583) -> (8.173577, 206.110954)
  line L2262 (8.173577, 206.110954) -> (7.461214, 206.110954)
  line L2263 (7.461214, 206.110954) -> (6.748177, 206.110954)
  line L2264 (6.748177, 206.110954) -> (6.750193, 206.609609)
  line L2265 (6.750193, 206.609609) -> (6.750194, 206.609611)
  point P0 (0, 0)
  constraints: 4532 end point
equation "\"d50\" = 2 * d49"
